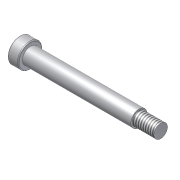
# Autodesk Inventor part: HW-00065
Saved by Autodesk Inventor 2012 (Build 160160000, 160)
## iProperties
Created: 2011-10-19
Part Number: HW-00065
Description: Shoulder Screw, .375 x 2.5" L, Alloy Steel
Document SubType Name: Modeling
Designer: dfoster
Density: 1 g/cm^3
Mass: 6.10398 g
Surface Area: 28.551 cm^2
Volume: 6.10398 cm^3
Material: Default
Title: Shoulder Screw, .375 x 2.5" L, Alloy Steel
Author: dfoster
Autodesk Inventor part; units mm, degrees
ref_plane "YZ Plane" through (0, 0, 0) normal (1, 0, 0) x (0, 1, 0)
ref_plane "XZ Plane" through (0, 0, 0) normal (0, 1, 0) x (-1, 0, 0)
ref_plane "XY Plane" through (0, 0, 0) normal (0, 0, 1) x (1, 0, 0)
sketch "Sketch1" plane through (0, 0, 0) normal (0, 0, 1) x (1, 0, 0)
  line L0 (0, 0) -> (0, 7.1437)
  line L1 (0, 7.1437) -> (6.35, 7.1438)
  line L2 (6.35, 7.1438) -> (6.35, 4.7625)
  line L3 (6.35, 4.7625) -> (69.85, 4.7625)
  line L4 (69.85, 4.7625) -> (69.85, 3.9688)
  line L5 (69.85, 3.9688) -> (82.55, 3.9688)
  line L6 (82.55, 3.9688) -> (82.55, 0)
  line L7 (82.55, 0) -> (0, 0)
  dimension "d0" = 7.1437
  dimension "d1" = 4.7625
  dimension "d2" = 3.9688
  dimension "d3" = 6.35
  dimension "d4" = 63.5
  dimension "d5" = 12.7
  constraints: 16 end point, 6 parallel, 1 perpendicular, 1 vertical
  measures "d0" distance between parallel lines of L7 L1
  measures "d1" distance between parallel lines of L7 L3
  measures "d2" distance between parallel lines of L7 L5
  measures "d3" distance of L0.end L1.end
  measures "d4" distance of L2.end L3.end
  measures "d5" distance of L4.end L5.end
revolve "Revolution1" add sketch "Sketch1" angle 360 about axis through (82.55, 0, 0) along (-1, 0, 0)
fillet "Fillet1" radius 0.508 2 edges at (0, -7.1437, 0) (6.35, -7.1437, 0)
thread "Thread1" size "5/16-18 UNC" class "2A" standard "ANSI Unified Screw Threads" full length
sketch "Sketch2" plane through (0, 0, 0) normal (-1, 0, 0) x (0, 0, 1)
  circle A0 centre (0, 0) radius 6.6357 projected
  line L0 (0, 2.7496) -> (2.3812, 1.3748)
  line L1 (2.3812, 1.3748) -> (2.3812, -1.3748)
  line L2 (2.3812, -1.3748) -> (0, -2.7496)
  line L3 (0, -2.7496) -> (-2.3813, -1.3748)
  line L4 (-2.3813, -1.3748) -> (-2.3813, 1.3748)
  line L5 (-2.3813, 1.3748) -> (0, 2.7496)
  dimension "d10" = 4.7625
  constraints: 12 end point, 1 coincident, 13 other
  measures "d10" distance between parallel lines of L0 L3
extrude "Extrusion1" cut sketch "Sketch2" against normal blind 3.175 contours L0 L1 L2 L3 L4 L5
body "Solid1"
